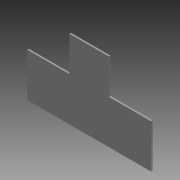
# Autodesk Inventor part: it top
Saved by Autodesk Inventor 2011 (Build 150239000, 239)
## iProperties
Created: 2011-09-03
Part Number: it top
Document SubType Name: Modeling
Designer: Matthew
Density: 1 g/cm^3
Author: Matthew
Autodesk Inventor part; units mm, degrees
ref_plane "YZ Plane" through (0, 0, 0) normal (1, 0, 0) x (0, 1, 0)
ref_plane "XZ Plane" through (0, 0, 0) normal (0, 1, 0) x (-1, 0, 0)
ref_plane "XY Plane" through (0, 0, 0) normal (0, 0, 1) x (1, 0, 0)
sketch "Sketch1" plane through (0, 0, 0) normal (0, 0, 1) x (1, 0, 0)
  line L0 (-37.7036, 22.272) -> (457.5964, 22.272)
  line L1 (457.5964, 22.272) -> (457.5964, -304.118)
  line L2 (457.5964, -304.118) -> (-37.7036, -304.118)
  line L3 (-37.7036, -304.118) -> (-37.7036, 22.272)
  point P0 (0, 0)
  dimension "d0" = 495.3
  dimension "d1" = 326.39
  constraints: 8 end point, 2 parallel, 1 horizontal, 1 perpendicular
  measures "d0" distance of L1.end L2.end
  measures "d1" distance of L0.end L1.end
extrude "Extrusion1" add sketch "Sketch1" along normal blind 6.35
sketch "Sketch2" plane through (0, 0, 6.35) normal (0, 0, 1) x (1, 0, 0)
  line L0 (-37.7036, 22.272) -> (457.5964, 22.272) projected
  line L1 (-37.7036, 22.272) -> (-18.6536, 22.272)
  line L2 (-18.6536, 22.272) -> (-18.6536, 15.922)
  line L3 (-18.6536, 15.922) -> (-37.7036, 15.922)
  line L4 (-37.7036, 15.922) -> (-37.7036, 22.272)
  line L5 (-18.6536, 15.922) -> (32.1464, 15.922)
  line L6 (32.1464, 15.922) -> (32.1464, 22.272)
  line L7 (32.1464, 22.272) -> (-18.6536, 22.272)
  line L8 (-18.6536, 22.272) -> (-18.6536, 15.922)
  line L9 (32.1464, 15.922) -> (82.9464, 15.922)
  line L10 (82.9464, 15.922) -> (82.9464, 22.272)
  line L11 (82.9464, 22.272) -> (32.1464, 22.272)
  line L12 (32.1464, 22.272) -> (32.1464, 15.922)
  line L13 (82.9464, 15.922) -> (133.7464, 15.922)
  line L14 (133.7464, 15.922) -> (133.7464, 22.272)
  line L15 (133.7464, 22.272) -> (82.9464, 22.272)
  line L16 (82.9464, 22.272) -> (82.9464, 15.922)
  line L17 (133.7464, 15.922) -> (184.5464, 15.922)
  line L18 (184.5464, 15.922) -> (184.5464, 22.272)
  line L19 (184.5464, 22.272) -> (133.7464, 22.272)
  line L20 (133.7464, 22.272) -> (133.7464, 15.922)
  line L21 (184.5464, 15.922) -> (235.3464, 15.922)
  line L22 (235.3464, 15.922) -> (235.3464, 22.272)
  line L23 (235.3464, 22.272) -> (184.5464, 22.272)
  line L24 (184.5464, 22.272) -> (184.5464, 15.922)
  line L25 (235.3464, 15.922) -> (286.1464, 15.922)
  line L26 (286.1464, 15.922) -> (286.1464, 22.272)
  line L27 (286.1464, 22.272) -> (235.3464, 22.272)
  line L28 (235.3464, 22.272) -> (235.3464, 15.922)
  line L29 (286.1464, 15.922) -> (336.9464, 15.922)
  line L30 (336.9464, 15.922) -> (336.9464, 22.272)
  line L31 (336.9464, 22.272) -> (286.1464, 22.272)
  line L32 (286.1464, 22.272) -> (286.1464, 15.922)
  line L33 (336.9464, 15.922) -> (387.7464, 15.922)
  line L34 (387.7464, 15.922) -> (387.7464, 22.272)
  line L35 (387.7464, 22.272) -> (336.9464, 22.272)
  line L36 (336.9464, 22.272) -> (336.9464, 15.922)
  line L37 (387.7464, 15.922) -> (438.5464, 15.922)
  line L38 (438.5464, 15.922) -> (438.5464, 22.272)
  line L39 (438.5464, 22.272) -> (387.7464, 22.272)
  line L40 (387.7464, 22.272) -> (387.7464, 15.922)
  line L41 (438.5464, 15.922) -> (457.5964, 15.922)
  line L42 (457.5964, 15.922) -> (457.5964, 22.272)
  line L43 (457.5964, 22.272) -> (438.5464, 22.272)
  line L44 (438.5464, 22.272) -> (438.5464, 15.922)
  point P0 (0, 0)
  dimension "d4" = 19.05
  dimension "d5" = 6.35
  dimension "d6" = 50.8
  dimension "d7" = 50.8
  dimension "d8" = 50.8
  dimension "d9" = 50.8
  dimension "d10" = 50.8
  dimension "d11" = 50.8
  dimension "d12" = 50.8
  dimension "d13" = 50.8
  dimension "d14" = 50.8
  constraints: 88 end point, 22 parallel, 11 horizontal, 11 perpendicular, 10 other
  measures "d4" distance of L2.end L3.end
  measures "d5" distance of L1.end L2.end
  measures "d6" distance of L7.end L6.end
  measures "d7" distance of L11.end L10.end
  measures "d8" distance of L15.end L14.end
  measures "d9" distance of L19.end L18.end
  measures "d10" distance of L23.end L22.end
  measures "d11" distance of L27.end L26.end
  measures "d12" distance of L31.end L30.end
  measures "d13" distance of L35.end L34.end
  measures "d14" distance of L39.end L38.end
extrude "Extrusion2" cut sketch "Sketch2" against normal blind 6.35 contours L0 L2 L3 L4 | L0 L10 L9 L6 | L0 L18 L17 L14 | L0 L26 L25 L22 | L0 L34 L33 L30 | L0 L42 L41 L38
sketch "Sketch3" plane through (0, 0, 6.35) normal (0, 0, 1) x (1, 0, 0)
  line L0 (457.5964, -304.118) -> (-37.7036, -304.118) projected
  line L1 (-37.7036, -304.118) -> (-18.6536, -304.118)
  line L2 (-18.6536, -304.118) -> (-18.6536, -297.768)
  line L3 (-18.6536, -297.768) -> (-37.7036, -297.768)
  line L4 (-37.7036, -297.768) -> (-37.7036, -304.118)
  line L5 (-18.6536, -297.768) -> (32.1464, -297.768)
  line L6 (32.1464, -297.768) -> (32.1464, -304.118)
  line L7 (32.1464, -304.118) -> (-18.6536, -304.118)
  line L8 (-18.6536, -304.118) -> (-18.6536, -297.768)
  line L9 (32.1464, -304.118) -> (82.9464, -304.118)
  line L10 (82.9464, -304.118) -> (82.9464, -297.768)
  line L11 (82.9464, -297.768) -> (32.1464, -297.768)
  line L12 (32.1464, -297.768) -> (32.1464, -304.118)
  line L13 (82.9464, -297.768) -> (133.7464, -297.768)
  line L14 (133.7464, -297.768) -> (133.7464, -304.118)
  line L15 (133.7464, -304.118) -> (82.9464, -304.118)
  line L16 (82.9464, -304.118) -> (82.9464, -297.768)
  line L17 (133.7464, -297.768) -> (184.5464, -297.768)
  line L18 (184.5464, -297.768) -> (184.5464, -304.118)
  line L19 (184.5464, -304.118) -> (133.7464, -304.118)
  line L20 (133.7464, -304.118) -> (133.7464, -297.768)
  line L21 (184.5464, -297.768) -> (235.3464, -297.768)
  line L22 (235.3464, -297.768) -> (235.3464, -304.118)
  line L23 (235.3464, -304.118) -> (184.5464, -304.118)
  line L24 (184.5464, -304.118) -> (184.5464, -297.768)
  line L25 (235.3464, -304.118) -> (286.1464, -304.118)
  line L26 (286.1464, -304.118) -> (286.1464, -297.768)
  line L27 (286.1464, -297.768) -> (235.3464, -297.768)
  line L28 (235.3464, -297.768) -> (235.3464, -304.118)
  line L29 (286.1464, -297.768) -> (336.9464, -297.768)
  line L30 (336.9464, -297.768) -> (336.9464, -304.118)
  line L31 (336.9464, -304.118) -> (286.1464, -304.118)
  line L32 (286.1464, -304.118) -> (286.1464, -297.768)
  line L33 (336.9464, -297.768) -> (387.7464, -297.768)
  line L34 (387.7464, -297.768) -> (387.7464, -304.118)
  line L35 (387.7464, -304.118) -> (336.9464, -304.118)
  line L36 (336.9464, -304.118) -> (336.9464, -297.768)
  line L37 (387.7464, -297.768) -> (438.5464, -297.768)
  line L38 (438.5464, -297.768) -> (438.5464, -304.118)
  line L39 (438.5464, -304.118) -> (387.7464, -304.118)
  line L40 (387.7464, -304.118) -> (387.7464, -297.768)
  line L41 (438.5464, -297.768) -> (457.5964, -297.768)
  line L42 (457.5964, -297.768) -> (457.5964, -304.118)
  line L43 (457.5964, -304.118) -> (438.5464, -304.118)
  line L44 (438.5464, -304.118) -> (438.5464, -297.768)
  point P0 (0, 0)
  dimension "d17" = 19.05
  dimension "d18" = 6.35
  constraints: 88 end point, 22 parallel, 11 horizontal, 11 perpendicular, 8 other
  measures "d17" distance of L3.end L2.end
  measures "d18" distance of L2.end L1.end
extrude "Extrusion3" cut sketch "Sketch3" against normal blind 6.35 contours L0 L38 L41 L42 | L0 L30 L33 L34 | L0 L14 L17 L18 | L0 L6 L11 L10 | L0 L4 L3 L2
sketch "Sketch4" plane through (0, 0, 6.35) normal (0, 0, 1) x (1, 0, 0)
  line L0 (336.9464, -304.118) -> (184.5464, -304.118) projected
  line L1 (184.5464, -304.118) -> (235.3464, -304.118)
  line L2 (235.3464, -304.118) -> (286.1464, -304.118)
  line L3 (286.1464, -304.118) -> (286.1464, -297.768)
  line L4 (286.1464, -297.768) -> (235.3464, -297.768)
  line L5 (235.3464, -297.768) -> (235.3464, -304.118)
  point P0 (0, 0)
  dimension "d21" = 50.8
  dimension "d22" = 50.8
  constraints: 10 end point, 2 parallel, 1 horizontal, 1 perpendicular, 1 point on line
  measures "d21" distance of L0.end L1.end
  measures "d22" distance of L4.end L3.end
extrude "Extrusion4" cut sketch "Sketch4" against normal blind 6.35
sketch "Sketch5" plane through (0, 0, 6.35) normal (0, 0, 1) x (1, 0, 0)
  line L0 (457.5964, 15.922) -> (457.5964, -297.768) projected
  line L1 (-37.7036, -297.768) -> (-37.7036, 15.922) projected
  line L2 (-37.7036, -297.768) -> (-18.6536, -297.768) projected
  line L3 (457.5964, 15.922) -> (457.5964, -166.323)
  line L4 (457.5964, -166.323) -> (451.2464, -166.323)
  line L5 (451.2464, -166.323) -> (451.2464, -115.523)
  line L6 (451.2464, -115.523) -> (457.5964, -115.523)
  line L7 (457.5964, -115.523) -> (457.5964, -166.323)
  line L8 (451.2464, -115.523) -> (457.5964, -115.523)
  line L9 (457.5964, -115.523) -> (457.5964, -64.723)
  line L10 (457.5964, -64.723) -> (451.2464, -64.723)
  line L11 (451.2464, -64.723) -> (451.2464, -115.523)
  line L12 (451.2464, -64.723) -> (457.5964, -64.723)
  line L13 (457.5964, -64.723) -> (457.5964, -13.923)
  line L14 (457.5964, -13.923) -> (451.2464, -13.923)
  line L15 (451.2464, -13.923) -> (451.2464, -64.723)
  line L16 (451.2464, -166.323) -> (457.5964, -166.323)
  line L17 (457.5964, -166.323) -> (457.5964, -217.123)
  line L18 (457.5964, -217.123) -> (451.2464, -217.123)
  line L19 (451.2464, -217.123) -> (451.2464, -166.323)
  line L20 (451.2464, -217.123) -> (457.5964, -217.123)
  line L21 (457.5964, -217.123) -> (457.5964, -267.923)
  line L22 (457.5964, -267.923) -> (451.2464, -267.923)
  line L23 (451.2464, -267.923) -> (451.2464, -217.123)
  line L24 (451.2464, -267.923) -> (457.5964, -267.923)
  line L25 (457.5964, -267.923) -> (457.5964, -297.768)
  line L26 (457.5964, -297.768) -> (451.2464, -297.768)
  line L27 (451.2464, -297.768) -> (451.2464, -267.923)
  line L28 (451.2464, -13.923) -> (457.5964, -13.923)
  line L29 (457.5964, -13.923) -> (457.5964, 15.922)
  line L30 (457.5964, 15.922) -> (451.2464, 15.922)
  line L31 (451.2464, 15.922) -> (451.2464, -13.923)
  line L32 (-37.7036, 15.922) -> (-31.3536, 15.922)
  line L33 (-31.3536, 15.922) -> (-31.3536, -13.923)
  line L34 (-31.3536, -13.923) -> (-37.7036, -13.923)
  line L35 (-37.7036, -13.923) -> (-37.7036, 15.922)
  line L36 (-37.7036, -64.723) -> (-31.3536, -64.723)
  line L37 (-31.3536, -64.723) -> (-31.3536, -115.523)
  line L38 (-31.3536, -115.523) -> (-37.7036, -115.523)
  line L39 (-37.7036, -115.523) -> (-37.7036, -64.723)
  line L40 (-37.7036, -166.323) -> (-31.3536, -166.323)
  line L41 (-31.3536, -166.323) -> (-31.3536, -217.123)
  line L42 (-31.3536, -217.123) -> (-37.7036, -217.123)
  line L43 (-37.7036, -217.123) -> (-37.7036, -166.323)
  line L44 (-37.7036, -267.923) -> (-31.3536, -267.923)
  line L45 (-31.3536, -267.923) -> (-31.3536, -297.768)
  line L46 (-31.3536, -297.768) -> (-37.7036, -297.768)
  line L47 (-37.7036, -297.768) -> (-37.7036, -267.923)
  point P0 (0, 0)
  dimension "d25" = 182.245
  dimension "d26" = 6.35
  dimension "d27" = 50.8
  dimension "d28" = 50.8
  dimension "d29" = 50.8
  dimension "d30" = 50.8
  dimension "d31" = 50.8
  dimension "d32" = 6.35
  constraints: 90 end point, 22 parallel, 11 horizontal, 11 perpendicular, 9 point on line
  measures "d25" distance of L0.start L3.end
  measures "d26" distance of L5.end L6.end
  measures "d27" distance of L4.end L5.end
  measures "d28" distance of L9.end L8.end
  measures "d29" distance of L13.end L12.end
  measures "d30" distance of L16.end L17.end
  measures "d31" distance of L20.end L21.end
  measures "d32" distance of L33.end L34.end
extrude "Extrusion5" cut sketch "Sketch5" against normal blind 6.35 contours L0 L14 L31 L30 | L0 L18 L19 L4 | L0 L26 L27 L22 | L1 L32 L33 L34 | L1 L36 L37 L38 | L1 L40 L41 L42 | L1 L44 L45 L2
sketch "Sketch6" plane through (0, 0, 6.35) normal (0, 0, 1) x (1, 0, 0)
  line L0 (457.5964, -13.923) -> (457.5964, -166.323) projected
  line L1 (457.5964, -13.923) -> (457.5964, -64.723)
  line L2 (457.5964, -64.723) -> (451.2464, -64.723)
  line L3 (451.2464, -64.723) -> (451.2464, -115.523)
  line L4 (451.2464, -115.523) -> (457.5964, -115.523)
  line L5 (457.5964, -115.523) -> (457.5964, -64.723)
  point P0 (0, 0)
  constraints: 10 end point, 2 parallel, 1 horizontal, 1 perpendicular, 1 point on line
extrude "Extrusion6" cut sketch "Sketch6" against normal blind 6.35
sketch "Sketch7" plane through (0, 0, 6.35) normal (0, 0, 1) x (1, 0, 0)
  line L0 (451.2464, -13.923) -> (451.2464, 15.922) projected
  line L1 (387.7464, 15.922) -> (336.9464, 15.922) projected
  line L2 (82.9464, 15.922) -> (32.1464, 15.922) projected
  line L3 (-31.3536, 15.922) -> (-31.3536, -13.923) projected
  line L4 (451.2464, -115.523) -> (451.2464, -64.723) projected
  line L5 (-31.3536, -6.7444) -> (44.8464, -6.7444)
  line L6 (44.8464, -6.7444) -> (44.8464, 15.922)
  line L7 (44.8464, 15.922) -> (44.8464, -60.278)
  line L8 (451.2464, -6.7444) -> (375.0464, -6.7444)
  line L9 (375.0464, -6.7444) -> (375.0464, 15.922)
  line L10 (375.0464, 15.922) -> (375.0464, -60.278)
  circle A0 centre (44.8464, -60.278) radius 25.4
  circle A1 centre (375.0464, -60.278) radius 25.4
  point P0 (0, 0)
  dimension "d37" = 76.2
  dimension "d38" = 76.2
  dimension "d39" = 76.2
  dimension "d40" = 76.2
  dimension "d41" = 50.8
  dimension "d42" = 50.8
  constraints: 12 end point, 4 perpendicular, 4 point on line, 2 centre point, 2 coincident, 2 collinear
  measures "d37" distance of L5.start L5.end
  measures "d38" distance of L6.end L7.end
  measures "d39" distance of L8.start L8.end
  measures "d40" distance of L9.end L10.end
  measures "d41" diameter of A0
  measures "d42" diameter of A1
extrude "Extrusion7" cut sketch "Sketch7" against normal blind 25.4
sketch "Sketch8" plane through (0, 0, 6.35) normal (0, 0, 1) x (1, 0, 0)
  circle A0 centre (44.8464, -60.278) radius 25.4 projected
  circle A1 centre (375.0464, -60.278) radius 25.4 projected
  point P0 (0, 0)
extrude "Extrusion8" add sketch "Sketch8" against normal blind 6.35
sketch "Sketch9" plane through (0, 0, 0) normal (0, 0, -1) x (-1, 0, 0)
  line L0 (-457.5964, -64.723) -> (-451.2464, -64.723) projected
  line L1 (-451.2464, -64.723) -> (-451.2464, -115.523) projected
  line L2 (-451.2464, -115.523) -> (-457.5964, -115.523) projected
  line L3 (-457.5964, -115.523) -> (-457.5964, -166.323) projected
  line L4 (-457.5964, -166.323) -> (-451.2464, -166.323) projected
  line L5 (-451.2464, -166.323) -> (-451.2464, -217.123) projected
  line L6 (-451.2464, -217.123) -> (-457.5964, -217.123) projected
  line L7 (-457.5964, -217.123) -> (-457.5964, -267.923) projected
  line L8 (-457.5964, -267.923) -> (-451.2464, -267.923) projected
  line L9 (-451.2464, -267.923) -> (-451.2464, -297.768) projected
  line L10 (-451.2464, -297.768) -> (-438.5464, -297.768) projected
  line L11 (-438.5464, -297.768) -> (-438.5464, -304.118) projected
  line L12 (-438.5464, -304.118) -> (-387.7464, -304.118) projected
  line L13 (-387.7464, -304.118) -> (-387.7464, -297.768) projected
  line L14 (-387.7464, -297.768) -> (-336.9464, -297.768) projected
  line L15 (-336.9464, -297.768) -> (-336.9464, -304.118) projected
  line L16 (-336.9464, -304.118) -> (-286.1464, -304.118) projected
  line L17 (-286.1464, -304.118) -> (-286.1464, -297.768) projected
  line L18 (-286.1464, -297.768) -> (-235.3464, -297.768) projected
  line L19 (-235.3464, -297.768) -> (-235.3464, -304.118) projected
  line L20 (-235.3464, -304.118) -> (-184.5464, -304.118) projected
  line L21 (-184.5464, -304.118) -> (-184.5464, -297.768) projected
  line L22 (-184.5464, -297.768) -> (-133.7464, -297.768) projected
  line L23 (-133.7464, -297.768) -> (-133.7464, -304.118) projected
  line L24 (-133.7464, -304.118) -> (-82.9464, -304.118) projected
  line L25 (-82.9464, -304.118) -> (-82.9464, -297.768) projected
  line L26 (-82.9464, -297.768) -> (-32.1464, -297.768) projected
  line L27 (-32.1464, -297.768) -> (-32.1464, -304.118) projected
  line L28 (-32.1464, -304.118) -> (18.6536, -304.118) projected
  line L29 (18.6536, -304.118) -> (18.6536, -297.768) projected
  line L30 (18.6536, -297.768) -> (31.3536, -297.768) projected
  line L31 (31.3536, -297.768) -> (31.3536, -267.923) projected
  line L32 (31.3536, -267.923) -> (37.7036, -267.923) projected
  line L33 (37.7036, -267.923) -> (37.7036, -217.123) projected
  line L34 (37.7036, -217.123) -> (31.3536, -217.123) projected
  line L35 (31.3536, -217.123) -> (31.3536, -166.323) projected
  line L36 (31.3536, -166.323) -> (37.7036, -166.323) projected
  line L37 (37.7036, -166.323) -> (37.7036, -115.523) projected
  line L38 (37.7036, -115.523) -> (31.3536, -115.523) projected
  line L39 (31.3536, -115.523) -> (31.3536, -64.723) projected
  line L40 (31.3536, -64.723) -> (37.7036, -64.723) projected
  line L41 (37.7036, -64.723) -> (37.7036, -13.923) projected
  line L42 (37.7036, -13.923) -> (31.3536, -13.923) projected
  line L43 (31.3536, -13.923) -> (31.3536, 15.922) projected
  line L44 (31.3536, 15.922) -> (18.6536, 15.922) projected
  line L45 (18.6536, 15.922) -> (18.6536, 22.272) projected
  line L46 (18.6536, 22.272) -> (-32.1464, 22.272) projected
  line L47 (-32.1464, 22.272) -> (-32.1464, 15.922) projected
  line L48 (-32.1464, 15.922) -> (-82.9464, 15.922) projected
  line L49 (-82.9464, 15.922) -> (-82.9464, 22.272) projected
  line L50 (-82.9464, 22.272) -> (-133.7464, 22.272) projected
  line L51 (-133.7464, 22.272) -> (-133.7464, 15.922) projected
  line L52 (-133.7464, 15.922) -> (-184.5464, 15.922) projected
  line L53 (-184.5464, 15.922) -> (-184.5464, 22.272) projected
  line L54 (-184.5464, 22.272) -> (-235.3464, 22.272) projected
  line L55 (-235.3464, 22.272) -> (-235.3464, 15.922) projected
  line L56 (-235.3464, 15.922) -> (-286.1464, 15.922) projected
  line L57 (-286.1464, 15.922) -> (-286.1464, 22.272) projected
  line L58 (-286.1464, 22.272) -> (-336.9464, 22.272) projected
  line L59 (-336.9464, 22.272) -> (-336.9464, 15.922) projected
  line L60 (-336.9464, 15.922) -> (-387.7464, 15.922) projected
  line L61 (-387.7464, 15.922) -> (-387.7464, 22.272) projected
  line L62 (-387.7464, 22.272) -> (-438.5464, 22.272) projected
  line L63 (-438.5464, 22.272) -> (-438.5464, 15.922) projected
  line L64 (-438.5464, 15.922) -> (-451.2464, 15.922) projected
  line L65 (-451.2464, 15.922) -> (-451.2464, -13.923) projected
  line L66 (-451.2464, -13.923) -> (-457.5964, -13.923) projected
  line L67 (-457.5964, -13.923) -> (-457.5964, -64.723) projected
  line L68 (18.6536, 15.922) -> (-438.5464, 15.922)
  point P0 (0, 0)
  constraints: 2 end point, 1 perpendicular
extrude "Extrusion9" cut sketch "Sketch9" against normal blind 25.4 contours L63 L62 L61 L68 | L59 L58 L57 L68 | L55 L54 L53 L68 | L51 L50 L49 L68 | L47 L46 L45 L68
sketch "Sketch10" plane through (0, 0, 0) normal (0, 0, -1) x (-1, 0, 0)
  line L0 (31.3536, 15.922) -> (-451.2464, 15.922) projected
  line L1 (-451.2464, 15.922) -> (-451.2464, -13.923) projected
  line L2 (-451.2464, -13.923) -> (-457.5964, -13.923) projected
  line L3 (-457.5964, -13.923) -> (-457.5964, -64.723) projected
  line L4 (-457.5964, -64.723) -> (-451.2464, -64.723) projected
  line L5 (-451.2464, -64.723) -> (-451.2464, -115.523) projected
  line L6 (-451.2464, -115.523) -> (-457.5964, -115.523) projected
  line L7 (-457.5964, -115.523) -> (-457.5964, -166.323) projected
  line L8 (-457.5964, -166.323) -> (-451.2464, -166.323) projected
  line L9 (-451.2464, -166.323) -> (-451.2464, -217.123) projected
  line L10 (-451.2464, -217.123) -> (-457.5964, -217.123) projected
  line L11 (-457.5964, -217.123) -> (-457.5964, -267.923) projected
  line L12 (-457.5964, -267.923) -> (-451.2464, -267.923) projected
  line L13 (-451.2464, -267.923) -> (-451.2464, -297.768) projected
  line L14 (-451.2464, -297.768) -> (-438.5464, -297.768) projected
  line L15 (-438.5464, -297.768) -> (-438.5464, -304.118) projected
  line L16 (-438.5464, -304.118) -> (-387.7464, -304.118) projected
  line L17 (-387.7464, -304.118) -> (-387.7464, -297.768) projected
  line L18 (-387.7464, -297.768) -> (-336.9464, -297.768) projected
  line L19 (-336.9464, -297.768) -> (-336.9464, -304.118) projected
  line L20 (-336.9464, -304.118) -> (-286.1464, -304.118) projected
  line L21 (-286.1464, -304.118) -> (-286.1464, -297.768) projected
  line L22 (-286.1464, -297.768) -> (-235.3464, -297.768) projected
  line L23 (-235.3464, -297.768) -> (-235.3464, -304.118) projected
  line L24 (-235.3464, -304.118) -> (-184.5464, -304.118) projected
  line L25 (-184.5464, -304.118) -> (-184.5464, -297.768) projected
  line L26 (-184.5464, -297.768) -> (-133.7464, -297.768) projected
  line L27 (-133.7464, -297.768) -> (-133.7464, -304.118) projected
  line L28 (-133.7464, -304.118) -> (-82.9464, -304.118) projected
  line L29 (-82.9464, -304.118) -> (-82.9464, -297.768) projected
  line L30 (-82.9464, -297.768) -> (-32.1464, -297.768) projected
  line L31 (-32.1464, -297.768) -> (-32.1464, -304.118) projected
  line L32 (-32.1464, -304.118) -> (18.6536, -304.118) projected
  line L33 (18.6536, -304.118) -> (18.6536, -297.768) projected
  line L34 (18.6536, -297.768) -> (31.3536, -297.768) projected
  line L35 (31.3536, -297.768) -> (31.3536, -267.923) projected
  line L36 (31.3536, -267.923) -> (37.7036, -267.923) projected
  line L37 (37.7036, -267.923) -> (37.7036, -217.123) projected
  line L38 (37.7036, -217.123) -> (31.3536, -217.123) projected
  line L39 (31.3536, -217.123) -> (31.3536, -166.323) projected
  line L40 (31.3536, -166.323) -> (37.7036, -166.323) projected
  line L41 (37.7036, -166.323) -> (37.7036, -115.523) projected
  line L42 (37.7036, -115.523) -> (31.3536, -115.523) projected
  line L43 (31.3536, -115.523) -> (31.3536, -64.723) projected
  line L44 (31.3536, -64.723) -> (37.7036, -64.723) projected
  line L45 (37.7036, -64.723) -> (37.7036, -13.923) projected
  line L46 (37.7036, -13.923) -> (31.3536, -13.923) projected
  line L47 (31.3536, -13.923) -> (31.3536, 15.922) projected
  line L48 (18.6536, -297.768) -> (-438.5464, -297.768)
  point P0 (0, 0)
  constraints: 2 end point, 1 perpendicular
extrude "Extrusion10" cut sketch "Sketch10" against normal blind 25.4 contours L33 L32 L31 L48 | L48 L17 L16 L15 | L29 L28 L27 L48 | L48 L21 L20 L19 | L25 L24 L23 L48
sketch "Sketch11" plane through (0, 0, 0) normal (0, 0, -1) x (-1, 0, 0)
  line L0 (37.7036, -297.768) -> (-457.5964, -297.768)
  line L1 (-457.5964, -297.768) -> (-457.5964, 15.922)
  line L2 (-457.5964, 15.922) -> (37.7036, 15.922)
  line L3 (37.7036, 15.922) -> (37.7036, -297.768)
  point P0 (0, 0)
  constraints: 8 end point, 2 parallel, 1 horizontal, 1 perpendicular
extrude "Extrusion11" add sketch "Sketch11" against normal blind 6.35
sketch "Sketch12" plane through (0, 0, 0) normal (0, 0, -1) x (-1, 0, 0)
  line L0 (37.7036, 15.922) -> (-457.5964, 15.922) projected
  line L1 (-457.5964, 15.922) -> (-457.5964, -297.768) projected
  line L2 (-457.5964, 15.922) -> (-457.5964, -123.778)
  line L3 (-457.5964, -123.778) -> (-289.1944, -123.778)
  line L4 (-289.1944, -123.778) -> (-289.1944, 15.922)
  line L5 (37.7036, 15.922) -> (-130.6984, 15.922)
  line L6 (-130.6984, 15.922) -> (-130.6984, -123.778)
  line L7 (-130.6984, -123.778) -> (37.7036, -123.778)
  line L8 (37.7036, -123.778) -> (37.7036, 15.922)
  point P0 (0, 0)
  dimension "d53" = 139.7
  dimension "d54" = 168.402
  dimension "d55" = 168.402
  dimension "d56" = 139.7
  constraints: 14 end point, 3 perpendicular, 2 parallel, 2 point on line, 1 horizontal
  measures "d53" distance of L0.end L2.end
  measures "d54" distance of L2.end L3.end
  measures "d55" distance of L7.end L6.end
  measures "d56" distance of L6.end L5.end
extrude "Extrusion12" cut sketch "Sketch12" against normal blind 25.4
sketch "Sketch13" plane through (0, 0, 0) normal (0, 0, -1) x (-1, 0, 0)
  line L0 (-130.6984, -123.778) -> (-130.6984, 15.922) projected
  line L1 (-130.6984, 15.922) -> (-289.1944, 15.922) projected
  line L2 (-289.1944, 15.922) -> (-289.1944, -123.778) projected
  line L3 (37.7036, -123.778) -> (37.7036, -297.768) projected
  line L4 (-130.6984, -123.778) -> (-289.1944, -123.778)
  point P0 (0, 0)
  constraints: 2 end point, 1 perpendicular
extrude "Extrusion13" cut sketch "Sketch13" against normal blind 25.4
body "Solid1"
